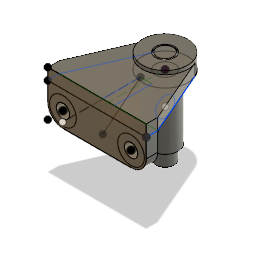
NOCTI Job 3 (Autodesk Fusion 360 design; units mm, degrees)
Autodesk Fusion 360 part; units mm, degrees
sketch "Sketch1" plane through (0, 0, 0) normal (0, 1, 0) x (1, 0, 0) in component "Component"
  line L0 (26.924, -11.049) -> (-26.924, -11.049)
  line L1 (-26.924, -11.049) -> (-26.924, 11.049)
  line L2 (-26.924, 11.049) -> (26.924, 11.049)
  line L3 (26.924, 11.049) -> (26.924, -11.049)
  line L4 (38.5464, -7.874) -> (-38.5464, -7.874)
  line L5 (-39.624, -6.7964) -> (-39.624, 6.7964)
  line L6 (-38.5464, 7.874) -> (38.5464, 7.874)
  line L7 (39.624, 6.7964) -> (39.624, -6.7964)
  line L8 (-39.624, 6.7964) -> (-39.624, -6.7964) construction
  line L9 (-39.624, 6.7964) -> (-38.5464, 7.874)
  line L10 (-39.624, 6.7964) -> (-38.1, 6.7964) construction
  line L11 (-39.624, -6.7964) -> (-38.5464, -7.874)
  line L12 (-39.624, -6.7964) -> (-38.1, -6.7964) construction
  line L13 (0, -1.75) -> (0, -22.5)
  line L14 (39.624, 6.7964) -> (38.5464, 7.874)
  line L15 (39.624, 6.7964) -> (39.624, -6.7964) construction
  line L16 (39.624, -6.7964) -> (38.5464, -7.874)
  line L17 (-45.72, 0) -> (46.9131, 0)
  dimension "d1" = 53.848
  dimension "d2" = 22.098
  dimension "d11" = 45
  dimension "d12" = 1.524
  dimension "d13" = 1.524
  dimension "d14" = 45
  constraint perpendicular L0 L1
  constraint parallel L0 L2
  constraint parallel L1 L3
  constraint horizontal L0
  constraint perpendicular L4 L5
  constraint parallel L4 L6
  constraint parallel L5 L7
  constraint horizontal L4
  constraint horizontal L10
  constraint horizontal L12
  constraint symmetric L5.end L13 L7.start
  constraint symmetric L6.start L13 L6.end
  constraint symmetric L5.start L13 L7.end
  constraint symmetric L4.end L13 L4.start
  constraint horizontal L17
  measures "d1" distance of L1.end L2.end
  measures "d2" distance of L0.end L1.end
  measures "d11" angle of L9 L10
  measures "d12" distance of L5.end L6.start
  measures "d13" distance of L5.start L4.end
  measures "d14" angle of L11 L12
revolve "Revolve1" add sketch "Sketch1" angle 360 about axis through (1.75, 0, 0) along (1, 0, 0) contours L1 L3 L6 L17 | L3 L6 L7 L14 L17 | L1 L2 L3 L6 | L1 L5 L6 L9 L17 makes body 1 in component "Component"
sketch "Sketch2" plane through (0, 0, 0) normal (0, 1, 0) x (1, 0, 0) in component "Component"
  circle A0 centre (0, 0) radius 8.001
  dimension "d16" = 16.002
  measures "d16" diameter of A0
sketch "Sketch1 (2)" plane through (0, 0, 0) normal (0, 1, 0) x (1, 0, 0) in component "Component'"
  circle A0 centre (0, 0) radius 8.001
  circle A1 centre (0, 0) radius 19.05
  line L0 (0, 0) -> (0, -57.15) construction
  line L1 (-41.275, -57.15) -> (41.275, -57.15)
  line L2 (-41.275, -57.15) -> (41.275, -57.15)
  line L3 (41.275, -57.15) -> (41.275, -47.498)
  line L4 (41.275, -47.498) -> (-41.275, -47.498)
  line L5 (-41.275, -47.498) -> (-41.275, -57.15)
  line L6 (-41.275, -47.498) -> (-17.4874, 7.5559)
  line L7 (41.275, -47.498) -> (17.4874, 7.5559)
  line L8 (4.826, -15.748) -> (-4.826, -15.748)
  line L9 (-4.826, -15.748) -> (-4.826, -47.498)
  line L10 (-4.826, -47.498) -> (4.826, -47.498)
  line L11 (4.826, -47.498) -> (4.826, -15.748)
  dimension "d17" = 16.002
  dimension "d18" = 38.1
  dimension "d19" = 57.15
  dimension "d21" = 82.55
  dimension "d22" = 9.652
  dimension "d39" = 9.652
  dimension "d40" = 31.75
  constraint coincident A0.centre A1.centre
  constraint concentric A0 A1
  constraint vertical L0
  constraint perpendicular L0 L1
  constraint midpoint L0.end L1
  constraint horizontal L2
  constraint vertical L3
  constraint horizontal L4
  constraint vertical L5
  constraint tangent A1 L7
  constraint tangent A1 L6
  constraint coincident A1 L6.end
  constraint coincident A1 L7.end
  constraint perpendicular L8 L9
  constraint parallel L8 L10
  constraint parallel L9 L11
  constraint horizontal L8
  constraint coincident L4 L10.end
  measures "d17" diameter of A0
  measures "d18" diameter of A1
  measures "d19" distance of A0.centre L0.end
  measures "d21" distance of L1.start L1.end
  measures "d22" distance of L1.start L4.end
  measures "d39" distance of L9.end L10.end
  measures "d40" distance of L8.end L9.end
extrude "Extrude1" add sketch "Sketch1 (2)" along normal blind 9.652 separate body contours A1 L4 L7 L11 | A1 L4 L9 L10 L11 | A1 L4 L6 L9 | L1 L2 L3 L4 L5 L10 makes body 2 in component "Component'"
extrude "Extrude2" add sketch "Sketch1 (2)" along normal blind 12.7 contours A1 L8 L9 L11 | A1 L8 L9 L11 bodies 2 in component "Component'"
sketch "Sketch2 (2)" plane through (0, 0, 57.15) normal (0, 0, 1) x (1, 0, 0) in component "Component'"
  line L0 (-41.275, 0) -> (41.275, 0)
  line L1 (41.275, 0) -> (41.275, 9.652)
  line L2 (41.275, 9.652) -> (-41.275, 9.652)
  line L3 (-41.275, 9.652) -> (-41.275, 0)
  line L4 (-41.275, 0) -> (41.275, 0)
  line L5 (-41.275, 9.652) -> (41.275, 9.652)
  line L6 (41.275, 9.652) -> (41.275, -15.748)
  line L7 (28.575, -28.448) -> (-28.575, -28.448)
  line L8 (-41.275, -15.748) -> (-41.275, 9.652)
  arc A0 (-41.275, -15.748) -> (-28.575, -28.448) centre (-28.575, -15.748) ccw
  arc A1 (28.575, -28.448) -> (41.275, -15.748) centre (28.575, -15.748) ccw
  circle A2 centre (-28.575, -15.748) radius 5.588
  circle A3 centre (-28.575, -15.748) radius 11.176
  circle A4 centre (28.575, -15.748) radius 5.588
  circle A5 centre (28.575, -15.748) radius 11.176
  point P0 (-41.275, -28.448)
  dimension "d28" = 82.55
  dimension "d44" = 82.55
  dimension "d45" = 38.1
  dimension "d46" = 12.7
  dimension "d47" = 12.7
  dimension "d48" = 11.176
  dimension "d49" = 22.352
  dimension "d50" = 11.176
  dimension "d51" = 22.352
  constraint horizontal L4
  constraint coincident L0.start L3.end
  constraint horizontal L5
  constraint vertical L6
  constraint horizontal L7
  constraint vertical L8
  constraint coincident L2.end L3.start
  constraint coincident P0 L7
  constraint coincident P0 L8
  constraint tangent L7 A0
  constraint tangent L8 A0
  constraint tangent L6 A1
  constraint tangent L7 A1
  constraint concentric A0 A2
  constraint concentric A2 A3
  constraint concentric A1 A4
  constraint concentric A4 A5
  measures "d28" distance of L0.start L0.end
  measures "d44" distance of L2.end L1.end
  measures "d45" distance of L2.end P0
  measures "d46" radius of A0
  measures "d47" radius of A1
  measures "d48" diameter of A2
  measures "d49" diameter of A3
  measures "d50" diameter of A4
  measures "d51" diameter of A5
extrude "Extrude6" add sketch "Sketch2 (2)" against normal blind 9.652 contours L0 L4 L6 L7 L8 A0 A1 bodies 2 in component "Component'"
extrude "Extrude7" add sketch "Sketch2 (2)" against normal up to surface (8.128 mm away) contours A3 | A5 bodies 2 in component "Component'"
extrude "Extrude8" add sketch "Sketch1 (2)" against normal up to surface (28.448 mm away) contours A1 L4 L9 L10 L11 | A1 L8 L9 L11 picked at (0, -16.8487) bodies 2 in component "Component'"
sketch "Sketch4" plane through (-4.826, 0, 0) normal (-1, 0, 0) x (0, 0, 1) in component "Component'"
  line L0 (15.748, -28.448) -> (47.498, -28.448)
  line L1 (47.498, -28.448) -> (47.498, 0)
  line L2 (47.498, 0) -> (15.748, 0)
  line L3 (15.748, 0) -> (15.748, -28.448)
  line L4 (15.748, 0) -> (47.498, -25.7106)
  line L5 (15.748, 0) -> (81.2963, 0) construction
  dimension "d58" = 39
  constraint horizontal L5
  constraint coincident L2.end L3.start
  constraint coincident L1 L4.end
  measures "d58" angle of L4 L5
extrude "Extrude10" cut sketch "Sketch4" against normal up to surface (9.652 mm away) contours L0 L1 L3 L4 bodies 2 in component "Component'"
fillet "Fillet1" radius 3.048 6 edges at (0, 0, 15.748) (-4.826, 0, 31.623) (-4.826, -12.8553, 47.498) (0, -25.7106, 47.498) (4.826, -12.8553, 47.498) (4.826, 0, 31.623) on bodies 2 in component "Component'"
fillet "Fillet1" radius 3.048 2 edges at (-23.0505, 0, 47.498) (23.0505, 0, 47.498) on bodies 2 in component "Component'"
component "Component" placed x (0, -1, 0) y (1, 0, 0) z (0, 0, 1) at (0, -26.924, 0)
component "Component'" placed x (1, 0, 0) y (0, 1, 0) z (0, 0, 1) at (0, 0, 0)
